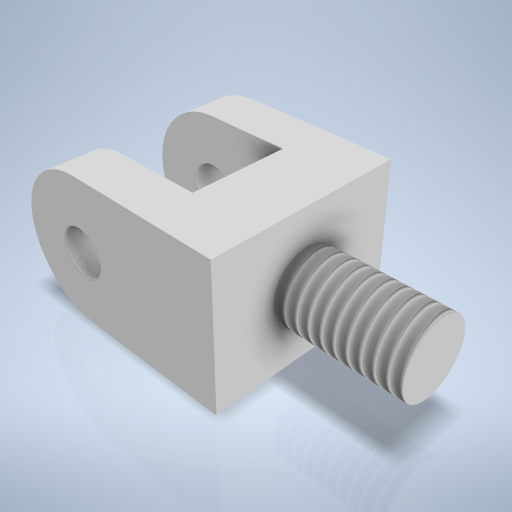
# Autodesk Inventor part: top_pleuel
Saved by Autodesk Inventor 2024.2 (Build 282272000, 272)
## iProperties
Created: 2024-05-15
Part Number: top_pleuel
Material: Generisch
Document SubType Name: Modeling
Designer: Fabri
Density: 1 g/cm^3
Appearance: Vorgabe
Author: Fabri
Autodesk Inventor part; units mm, degrees
ref_plane "YZ Plane" through (0, 0, 0) normal (1, 0, 0) x (0, 1, 0)
ref_plane "XZ Plane" through (0, 0, 0) normal (0, 1, 0) x (-1, 0, 0)
ref_plane "XY Plane" through (0, 0, 0) normal (0, 0, 1) x (1, 0, 0)
sketch "Skizze1" plane through (0, 0, 0) normal (0, 1, 0) x (-1, 0, 0)
  line L0 (0, 3) -> (9.5, 3)
  line L1 (9.5, 3) -> (9.5, -3)
  line L2 (9.5, -3) -> (0, -3)
  line L3 (0, -3) -> (0, 3)
  point P0 (0, 0)
  point P1 (0, 0)
  dimension "d0" = 6
  dimension "d1" = 9.5
  constraints: 8 end point, 2 parallel, 1 coincident, 1 horizontal, 1 midpoint, 1 perpendicular
  measures "d0" distance between parallel lines of L2 L0
  measures "d1" distance between parallel lines of L3 L1
extrude "Extrusion1" add sketch "Skizze1" along normal blind 8
fillet "Rundung1" radius 3 2 edges at (-9.5, 4, -3) (-9.5, 4, 3)
sketch "Skizze5" plane through (0, 8, 0) normal (0, 1, 0) x (1, 0, 0)
  arc A0 (-6.5, 3) -> (-6.5, -3) centre (-6.5, 0) ccw projected
  point P0 (0, 0)
  constraints: 1 coincident
hole "Bohrung2" at (-6.5, 8, 0) direction (0, -1, 0) diameter 2 depth 8
sketch "Skizze3" plane through (0, 0, -3) normal (0, 0, -1) x (-1, 0, 0)
  line L0 (3, 6) -> (11.5, 6)
  line L1 (11.5, 6) -> (11.5, 2)
  line L2 (11.5, 2) -> (3, 2)
  line L3 (3, 2) -> (3, 6)
  line L4 (9.5, 0) -> (9.5, 8) projected
  line L5 (0, 0) -> (0, 8) projected
  point P0 (3, 4)
  point P1 (0, 4)
  point P2 (7.25, 2)
  point P3 (11.5, 4)
  dimension "d12" = 6.5
  dimension "d13" = 4
  dimension "d14" = 2
  constraints: 8 end point, 4 midpoint, 2 parallel, 1 horizontal, 1 horizontal alignment, 1 perpendicular
  measures "d12" distance between parallel lines of L3 L4
  measures "d13" distance from line of point (7.25, 2) L0
  measures "d14" distance from line of L4 point (11.5, 4)
extrude "Extrusion2" cut sketch "Skizze3" against normal up to surface (6 mm away)
sketch "Skizze4" plane through (0, 0, 3) normal (1, 0, 0) x (0, 0, -1)
  circle A0 centre (3, 4) radius 1.5
  line L0 (6, 0) -> (6, 8) projected
  line L1 (0, 0) -> (6, 0) projected
  point P0 (3, 0)
  point P1 (6, 4)
  point P2 (3, 0)
  dimension "d17" = 3
  constraints: 2 midpoint, 1 centre point, 1 horizontal alignment, 1 vertical alignment
  measures "d17" diameter of A0
extrude "Extrusion3" add sketch "Skizze4" along normal blind 5
thread "Gewinde1" size "M3x0.5" class "6g" standard "ISO Metric profile" length 18
